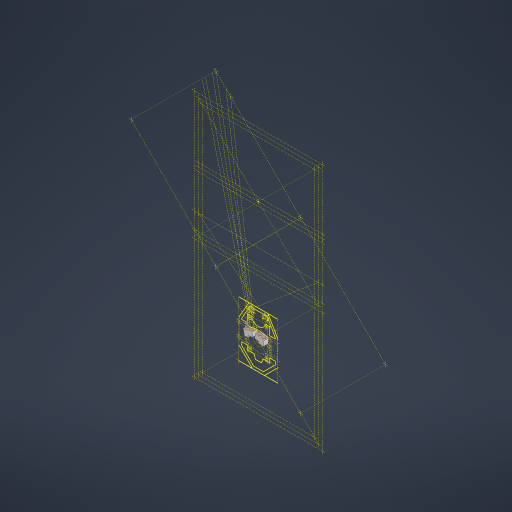
# Autodesk Inventor part: sensormount-2
Saved by Autodesk Inventor 2023.5 (Build 275446000, 446)
## iProperties
Created: 2025-01-19
Part Number: sensormount-2
Material: 一般
Document SubType Name: Modeling
Designer: IshiiLabHonda
Density: 1 g/cm^3
Appearance: 既定
Author: IshiiLabHonda
Autodesk Inventor part; units mm, degrees
(part 1 of 2)
ref_plane "YZ Plane" through (0, 0, 0) normal (1, 0, 0) x (0, 1, 0)
ref_plane "XZ Plane" through (0, 0, 0) normal (0, 1, 0) x (-1, 0, 0)
ref_plane "XY Plane" through (0, 0, 0) normal (0, 0, 1) x (1, 0, 0)
derived "chassis.ipt"
sketch "スケッチ1" plane through (0, 0, 0) normal (0, 0, 1) x (1, 0, 0)
  line L0 (-90, 90) -> (90, 90) construction
  line L1 (90, 90) -> (90, -90) construction
  line L2 (90, -90) -> (-90, -90) construction
  line L3 (-90, -90) -> (-90, 90) construction
  line L4 (-90, 90) -> (-90, 270) construction
  line L5 (-90, 270) -> (90, 270) construction
  line L6 (90, 270) -> (90, 90) construction
  line L7 (-90, 90) -> (90, -90) construction
  line L8 (90, 90) -> (-90, -90) construction
  line L9 (0, 0) -> (0, 10) construction
  line L10 (0, 0) -> (10, 0) construction
  line L11 (-90, 270) -> (90, 90) construction
  line L12 (-90, 90) -> (90, 270) construction
  line L13 (-96, 276) -> (96, 276) construction
  line L14 (96, 276) -> (96, -96) construction
  line L15 (96, -96) -> (-96, -96) construction
  line L16 (-96, -96) -> (-96, 276) construction
  line L17 (-84, 264) -> (84, 264) construction
  line L18 (84, 264) -> (84, -84) construction
  line L19 (84, -84) -> (-84, -84) construction
  line L20 (-84, -84) -> (-84, 264) construction
  line L21 (-96, 96) -> (96, 96) construction
  line L22 (-96, 84) -> (96, 84) construction
  line L23 (-63.6396, 63.6396) -> (63.6396, 190.9188) construction
  line L24 (63.6396, 190.9188) -> (190.9188, 63.6396) construction
  line L25 (190.9188, 63.6396) -> (63.6396, -63.6396) construction
  line L26 (63.6396, -63.6396) -> (-63.6396, 63.6396) construction
  line L27 (-190.9188, 190.9188) -> (-63.6396, 318.1981) construction
  line L28 (-63.6396, 318.1981) -> (63.6396, 190.9188) construction
  line L29 (-63.6396, 63.6396) -> (-190.9188, 190.9188) construction
  line L30 (-96, 120) -> (96, 120) construction
  line L31 (-96, 186) -> (96, 186) construction
  line L32 (-96, 174) -> (96, 174) construction
  line L33 (-96, 180) -> (96, 180) construction
  point P0 (-63.6396, 318.1981)
  point P1 (-90, 120)
  point P2 (90, 120)
  point P3 (0, 180)
sketch "スケッチ2" plane through (0, 0, 0) normal (0, 0, 1) x (1, 0, 0)
  line L0 (63.6396, 190.9188) -> (190.9188, 63.6396) construction
  line L1 (-63.6396, 318.1981) -> (63.6396, 190.9188) construction
  line L2 (-84, 264) -> (84, 264) construction
  line L3 (-90, 270) -> (90, 270) construction
  line L4 (90, 270) -> (90, 90) construction
  line L5 (-96, 276) -> (96, 276) construction
  line L6 (-90, 90) -> (90, 270) construction
  line L7 (-90, 270) -> (90, 90) construction
  line L8 (-63.6396, 63.6396) -> (63.6396, 190.9188) construction
  line L9 (-96, 120) -> (96, 120) construction
  line L10 (-90, 90) -> (90, 90) construction
  line L11 (-96, 96) -> (96, 96) construction
  line L12 (-96, 84) -> (96, 84) construction
  line L13 (90, -90) -> (-90, -90) construction
  line L14 (0, 0) -> (0, 10) construction
  line L15 (0, 0) -> (10, 0) construction
  line L16 (190.9188, 63.6396) -> (63.6396, -63.6396) construction
  line L17 (63.6396, -63.6396) -> (-63.6396, 63.6396) construction
  line L18 (84, -84) -> (-84, -84) construction
  line L19 (96, -96) -> (-96, -96) construction
  line L20 (-90, 90) -> (-90, 270) construction
  line L21 (-63.6396, 63.6396) -> (-190.9188, 190.9188) construction
  line L22 (-190.9188, 190.9188) -> (-63.6396, 318.1981) construction
  line L23 (96, 276) -> (96, -96) construction
  line L24 (-96, -96) -> (-96, 276) construction
  line L25 (84, 264) -> (84, -84) construction
  line L26 (-84, -84) -> (-84, 264) construction
  line L27 (90, 90) -> (90, -90) construction
  line L28 (-90, 90) -> (90, -90) construction
  line L29 (90, 90) -> (-90, -90) construction
  line L30 (-90, -90) -> (-90, 90) construction
  circle A0 centre (0, 0) radius 16 construction
  circle A1 centre (0, 0) radius 7.5 construction
  line L31 (20, 11.5) -> (28.75, 11.5) construction
  line L32 (28.75, 11.5) -> (28.75, -11.5) construction
  line L33 (28.75, -11.5) -> (20, -11.5) construction
  line L34 (20, -11.5) -> (20, 11.5) construction
  line L35 (20, 11.5) -> (18, 11.5) construction
  line L36 (18, 11.5) -> (18, -11.5) construction
  line L37 (18, -11.5) -> (20, -11.5) construction
  line L38 (18, 1.5) -> (17, 1.5) construction
  line L39 (17, -1.5) -> (18, -1.5) construction
  line L40 (-17, 26) -> (17, 26) construction
  line L41 (17, 26) -> (17, -20) construction
  line L42 (17, -20) -> (-17, -20) construction
  line L43 (-17, -20) -> (-17, 26) construction
  line L44 (-20, 11.5) -> (-18, 11.5) construction
  line L45 (-17, -1.5) -> (-18, -1.5) construction
  line L46 (-20, -11.5) -> (-20, 11.5) construction
  line L47 (-18, 11.5) -> (-18, -11.5) construction
  line L48 (-28.75, -11.5) -> (-20, -11.5) construction
  line L49 (-20, 11.5) -> (-28.75, 11.5) construction
  line L50 (-28.75, 11.5) -> (-28.75, -11.5) construction
  line L51 (-18, -11.5) -> (-20, -11.5) construction
  line L52 (-18, 1.5) -> (-17, 1.5) construction
  line L53 (-14.5, 26) -> (-14.5, -20) construction
  line L54 (14.5, 26) -> (14.5, -20) construction
  line L55 (-10.5, 26) -> (-10.5, 21) construction
  line L56 (-10.5, 21) -> (-14.5, 21) construction
  line L57 (-14.5, 26) -> (-10.5, 21) construction
  line L58 (-10.5, 26) -> (-14.5, 21) construction
  circle A2 centre (-12.5, 23.5) radius 1 construction
  line L59 (10.5, 26) -> (10.5, 21) construction
  line L60 (10.5, 21) -> (14.5, 21) construction
  line L61 (10.5, 26) -> (14.5, 21) construction
  line L62 (10.5, 21) -> (14.5, 26) construction
  circle A3 centre (12.5, 23.5) radius 1 construction
  line L63 (-14.5, -15) -> (-10.5, -15) construction
  line L64 (-10.5, -15) -> (-10.5, -20) construction
  line L65 (10.5, -20) -> (10.5, -15) construction
  line L66 (10.5, -15) -> (14.5, -15) construction
  line L67 (-14.5, -15) -> (-10.5, -20) construction
  line L68 (-10.5, -15) -> (-14.5, -20) construction
  circle A4 centre (-12.5, -17.5) radius 1 construction
  line L69 (10.5, -15) -> (14.5, -20) construction
  line L70 (14.5, -15) -> (10.5, -20) construction
  circle A5 centre (12.5, -17.5) radius 1 construction
  point P0 (90, 120)
  point P1 (-90, 120)
  point P2 (-63.6396, 318.1981)
  point P3 (-12.5, -17.5)
sketch "スケッチ3" plane through (0, 0, 0) normal (0, 0, 1) x (1, 0, 0)
  line L0 (63.6396, 190.9188) -> (190.9188, 63.6396) construction
  line L1 (-63.6396, 318.1981) -> (63.6396, 190.9188) construction
  line L2 (-84, 264) -> (84, 264) construction
  line L3 (-90, 270) -> (90, 270) construction
  line L4 (90, 270) -> (90, 90) construction
  line L5 (-96, 276) -> (96, 276) construction
  line L6 (-90, 90) -> (90, 270) construction
  line L7 (-90, 270) -> (90, 90) construction
  line L8 (-63.6396, 63.6396) -> (63.6396, 190.9188) construction
  line L9 (-96, 120) -> (96, 120) construction
  line L10 (-90, 90) -> (90, 90) construction
  line L11 (-96, 96) -> (96, 96) construction
  line L12 (-96, 84) -> (96, 84) construction
  line L13 (90, -90) -> (-90, -90) construction
  line L14 (0, 0) -> (0, 10) construction
  line L15 (0, 0) -> (10, 0) construction
  line L16 (190.9188, 63.6396) -> (63.6396, -63.6396) construction
  line L17 (63.6396, -63.6396) -> (-63.6396, 63.6396) construction
  line L18 (84, -84) -> (-84, -84) construction
  line L19 (96, -96) -> (-96, -96) construction
  line L20 (-90, 90) -> (-90, 270) construction
  line L21 (-63.6396, 63.6396) -> (-190.9188, 190.9188) construction
  line L22 (-190.9188, 190.9188) -> (-63.6396, 318.1981) construction
  line L23 (96, 276) -> (96, -96) construction
  line L24 (-96, -96) -> (-96, 276) construction
  line L25 (84, 264) -> (84, -84) construction
  line L26 (-84, -84) -> (-84, 264) construction
  line L27 (90, 90) -> (90, -90) construction
  line L28 (-90, 90) -> (90, -90) construction
  line L29 (90, 90) -> (-90, -90) construction
  line L30 (-90, -90) -> (-90, 90) construction
  line L31 (-18, 1.5) -> (-17, 1.5) construction
  line L32 (-17, -1.5) -> (-18, -1.5) construction
  line L33 (-20, 11.5) -> (-18, 11.5) construction
  line L34 (-28.75, 11.5) -> (-28.75, -11.5) construction
  line L35 (63.6396, -63.6396) -> (-63.6396, 63.6396) construction
  line L36 (84, -84) -> (-84, -84) construction
  line L37 (-90, -90) -> (-90, 90) construction
  line L38 (96, -96) -> (-96, -96) construction
  line L39 (-90, 90) -> (90, 90) construction
  line L40 (90, -90) -> (-90, -90) construction
  line L41 (90, 90) -> (-90, -90) construction
  line L42 (-90, 90) -> (90, -90) construction
  line L43 (90, 90) -> (90, -90) construction
  line L44 (-28.75, -11.5) -> (-20, -11.5) construction
  line L45 (-20, 11.5) -> (-28.75, 11.5) construction
  line L46 (-18, 11.5) -> (-18, -11.5) construction
  line L47 (-18, -11.5) -> (-20, -11.5) construction
  line L48 (0, 0) -> (0, 10) construction
  line L49 (0, 0) -> (10, 0) construction
  circle A0 centre (0, 0) radius 16 construction
  circle A1 centre (0, 0) radius 7.5 construction
  line L50 (-14.5, 26) -> (-14.5, -20) construction
  line L51 (-17, 26) -> (17, 26) construction
  line L52 (-17, -20) -> (-17, 26) construction
  line L53 (17, -20) -> (-17, -20) construction
  line L54 (-14.5, -15) -> (-10.5, -15) construction
  circle A2 centre (-12.5, -17.5) radius 1 construction
  line L55 (-10.5, -15) -> (-14.5, -20) construction
  line L56 (-14.5, -15) -> (-10.5, -20) construction
  line L57 (-63.6396, 318.1981) -> (63.6396, 190.9188) construction
  line L58 (-84, 264) -> (84, 264) construction
  line L59 (-90, 270) -> (90, 270) construction
  line L60 (90, 270) -> (90, 90) construction
  line L61 (-96, 276) -> (96, 276) construction
  line L62 (-90, 90) -> (90, 270) construction
  line L63 (-90, 270) -> (90, 90) construction
  line L64 (-63.6396, 63.6396) -> (63.6396, 190.9188) construction
  line L65 (-96, 120) -> (96, 120) construction
  line L66 (-96, 96) -> (96, 96) construction
  line L67 (-96, 84) -> (96, 84) construction
  line L68 (84, 264) -> (84, -84) construction
  line L69 (96, 276) -> (96, -96) construction
  line L70 (-96, -96) -> (-96, 276) construction
  line L71 (-84, -84) -> (-84, 264) construction
  line L72 (-63.6396, 63.6396) -> (-190.9188, 190.9188) construction
  line L73 (-90, 90) -> (-90, 270) construction
  line L74 (-190.9188, 190.9188) -> (-63.6396, 318.1981) construction
  line L75 (-20, -11.5) -> (-20, 11.5) construction
  line L76 (10.5, -15) -> (14.5, -15) construction
  line L77 (10.5, -20) -> (10.5, -15) construction
  circle A3 centre (12.5, -17.5) radius 1 construction
  line L78 (10.5, -15) -> (14.5, -20) construction
  line L79 (14.5, -15) -> (10.5, -20) construction
  line L80 (-10.5, -15) -> (-10.5, -20) construction
  line L81 (63.6396, 190.9188) -> (190.9188, 63.6396) construction
  line L82 (190.9188, 63.6396) -> (63.6396, -63.6396) construction
  line L83 (20, 11.5) -> (28.75, 11.5) construction
  line L84 (28.75, 11.5) -> (28.75, -11.5) construction
  line L85 (17, -1.5) -> (18, -1.5) construction
  line L86 (18, -11.5) -> (20, -11.5) construction
  line L87 (28.75, -11.5) -> (20, -11.5) construction
  line L88 (14.5, 26) -> (14.5, -20) construction
  line L89 (17, 26) -> (17, -20) construction
  line L90 (18, 11.5) -> (18, -11.5) construction
  line L91 (20, -11.5) -> (20, 11.5) construction
  line L92 (20, 11.5) -> (18, 11.5) construction
  line L93 (18, 1.5) -> (17, 1.5) construction
  line L94 (-10.5, 26) -> (-10.5, 21) construction
  line L95 (10.5, 21) -> (14.5, 21) construction
  circle A4 centre (12.5, 23.5) radius 1 construction
  line L96 (10.5, 26) -> (14.5, 21) construction
  line L97 (10.5, 21) -> (14.5, 26) construction
  line L98 (10.5, 26) -> (10.5, 21) construction
  line L99 (-10.5, 21) -> (-14.5, 21) construction
  circle A5 centre (-12.5, 23.5) radius 1 construction
  line L100 (-14.5, 26) -> (-10.5, 21) construction
  line L101 (-10.5, 26) -> (-14.5, 21) construction
  line L102 (29.25, 41.8164) -> (29.25, -41.1836) construction
  line L103 (29.25, -41.1836) -> (-29.25, -41.1836) construction
  line L104 (-29.25, -41.1836) -> (-29.25, 41.8164) construction
  line L105 (-29.25, 8.5) -> (-17, 8.5) construction
  line L106 (-17, 8.5) -> (-17, -8.5) construction
  line L107 (-17, -8.5) -> (-29.25, -8.5) construction
  line L108 (29.25, 8.5) -> (17, 8.5) construction
  line L109 (17, 8.5) -> (17, -8.5) construction
  line L110 (17, -8.5) -> (29.25, -8.5) construction
  line L111 (-2.6232, 12.9386) -> (-1.1431, 4.3146) construction
  line L112 (6.5255, 35.7419) -> (9.7395, 39.5722) construction
  line L113 (5.3082, 35.458) -> (9.8077, 40.8203) construction
  line L114 (10.2875, 31.2799) -> (5.3082, 35.458) construction
  line L115 (9.8077, 40.8203) -> (10.2875, 31.2799) construction
  line L116 (10.3558, 32.528) -> (9.7395, 39.5722) construction
  line L117 (10.3558, 32.528) -> (6.5255, 35.7419) construction
  line L118 (10.2875, 31.2799) -> (12.5856, 29.3515) construction
  line L119 (9.7395, 39.5722) -> (13.5697, 36.3582) construction
  line L120 (6.5255, 35.7419) -> (13.5697, 36.3582) construction
  line L121 (13.5697, 36.3582) -> (10.3558, 32.528) construction
  line L122 (5.3082, 35.458) -> (14.787, 36.6422) construction
  line L123 (9.8077, 40.8203) -> (14.787, 36.6422) construction
  line L124 (14.787, 36.6422) -> (10.2875, 31.2799) construction
  line L125 (12.5856, 29.3515) -> (17.0851, 34.7138) construction
  line L126 (17.0851, 34.7138) -> (14.787, 36.6422) construction
  line L127 (-3.4819, 12.0302) -> (-2.6362, 7.1023) construction
  line L128 (-8.4099, 11.1845) -> (-2.6362, 7.1023) construction
  line L129 (-7.5641, 6.2565) -> (-3.4819, 12.0302) construction
  line L130 (-9.0295, 11.8391) -> (-2.6232, 12.9386) construction
  line L131 (-7.5641, 6.2565) -> (-8.4099, 11.1845) construction
  line L132 (-1.1431, 4.3146) -> (-7.5495, 3.2152) construction
  line L133 (-7.5495, 3.2152) -> (-9.0295, 11.8391) construction
  line L134 (-63.6396, 318.1981) -> (-5.523, 9.1434) construction
  line L135 (10.0476, 36.0501) -> (-90, 120) construction
  line L136 (-5.523, 9.1434) -> (-79.4519, 302.3857) construction
  line L137 (-5.523, 9.1434) -> (-41.5159, 296.0744) construction
  line L138 (-10.0476, 36.0501) -> (90, 120) construction
  line L139 (-9.7395, 39.5722) -> (-6.5255, 35.7419) construction
  line L140 (-9.8077, 40.8203) -> (-5.3082, 35.458) construction
  line L141 (-14.787, 36.6422) -> (-9.8077, 40.8203) construction
  line L142 (-5.3082, 35.458) -> (-14.787, 36.6422) construction
  line L143 (-13.5697, 36.3582) -> (-6.5255, 35.7419) construction
  line L144 (-13.5697, 36.3582) -> (-9.7395, 39.5722) construction
  line L145 (-14.787, 36.6422) -> (-17.0851, 34.7138) construction
  line L146 (-6.5255, 35.7419) -> (-10.3558, 32.528) construction
  line L147 (-9.7395, 39.5722) -> (-10.3558, 32.528) construction
  line L148 (-9.8077, 40.8203) -> (-10.2875, 31.2799) construction
  line L149 (-5.3082, 35.458) -> (-10.2875, 31.2799) construction
  line L150 (-10.2875, 31.2799) -> (-14.787, 36.6422) construction
  line L151 (-17.0851, 34.7138) -> (-12.5856, 29.3515) construction
  line L152 (-12.5856, 29.3515) -> (-10.2875, 31.2799) construction
  line L153 (-10.3558, 32.528) -> (-13.5697, 36.3582) construction
  circle A6 centre (-6.8337, 32.2199) radius 0.625 construction
  circle A7 centre (-6.8337, 32.2199) radius 0.8 construction
  circle A8 centre (-6.8337, 32.2199) radius 1.5 construction
  circle A9 centre (-13.6863, 32.9968) radius 1.5 construction
  circle A10 centre (-13.6863, 32.9968) radius 0.8 construction
  circle A11 centre (-13.6863, 32.9968) radius 0.625 construction
  line L154 (-2.6362, 7.1023) -> (-7.5641, 6.2565) construction
  line L155 (-7.9301, 5.4327) -> (-1.5237, 6.5322) construction
  line L156 (-7.987, 8.7205) -> (-3.059, 9.5662) construction
  line L157 (-4.5927, 3.7226) -> (-5.1001, 6.6794) construction
  line L158 (-8.4099, 11.1845) -> (-3.4819, 12.0302) construction
  circle A12 centre (13.6863, 32.9968) radius 1.5 construction
  circle A13 centre (13.6863, 32.9968) radius 0.625 construction
  circle A14 centre (13.6863, 32.9968) radius 0.8
  circle A15 centre (6.8337, 32.2199) radius 1.5 construction
  circle A16 centre (6.8337, 32.2199) radius 0.8
  circle A17 centre (6.8337, 32.2199) radius 0.625 construction
  line L159 (-29.25, -41.1836) -> (29.25, -41.1836)
  line L160 (-29.25, 41.8164) -> (29.25, 41.8164)
  line L161 (-10.0476, 36.0501) -> (-6.8337, 32.2199) construction
  line L162 (-29.25, 15.7886) -> (-14.2228, 41.8164)
  line L163 (-29.25, -20.8975) -> (-8.9639, -41.1836)
  line L164 (29.25, 15.7886) -> (14.2228, 41.8164)
  line L165 (29.25, -20.8975) -> (8.9639, -41.1836)
  line L166 (25.25, 15.774) -> (25.25, 14.5)
  line L167 (25.25, 14.5) -> (17, 14.5)
  line L168 (3.695, 18.0905) -> (-3.695, 18.0905)
  line L169 (-17, 14.5) -> (-25.25, 14.5)
  line L170 (-25.25, 14.5) -> (-25.25, 15.774)
  line L171 (1.1431, 4.3146) -> (7.5495, 3.2152) construction
  line L172 (7.5495, 3.2152) -> (9.0295, 11.8391) construction
  line L173 (2.6232, 12.9386) -> (1.1431, 4.3146) construction
  line L174 (2.6362, 7.1023) -> (7.5641, 6.2565) construction
  line L175 (7.9301, 5.4327) -> (1.5237, 6.5322) construction
  line L176 (8.4099, 11.1845) -> (2.6362, 7.1023) construction
  line L177 (7.5641, 6.2565) -> (3.4819, 12.0302) construction
  line L178 (3.4819, 12.0302) -> (2.6362, 7.1023) construction
  line L179 (8.4099, 11.1845) -> (3.4819, 12.0302) construction
  line L180 (7.5641, 6.2565) -> (8.4099, 11.1845) construction
  line L181 (9.0295, 11.8391) -> (2.6232, 12.9386) construction
  line L182 (-9.7365, 22.9366) -> (-9.7365, 26)
  line L183 (9.7365, 22.9366) -> (9.7365, 26)
  line L184 (9.7365, 26) -> (17, 26)
  line L185 (17, 26) -> (17, 14.5)
  line L186 (-9.7365, 26) -> (-17, 26)
  line L187 (-17, 26) -> (-17, 14.5)
  line L188 (-9.7365, 22.9366) -> (-3.695, 18.0905)
  line L189 (9.7365, 22.9366) -> (3.695, 18.0905)
  line L190 (-17, -14.5) -> (-25.25, -14.5)
  line L191 (-25.25, -14.5) -> (-25.25, -19.2406)
  line L192 (-25.25, -19.2406) -> (-7.307, -37.1836)
  line L193 (-7.307, -37.1836) -> (7.307, -37.1836)
  line L194 (7.307, -37.1836) -> (25.25, -19.2406)
  line L195 (25.25, -19.2406) -> (25.25, -14.5)
  line L196 (25.25, -14.5) -> (17, -14.5)
  line L197 (17, -14.5) -> (17, -20.8804)
  line L198 (17, -20.8804) -> (6.6466, -20.8804)
  line L199 (6.6466, -20.8804) -> (4.5158, -27.0126)
  line L200 (4.5158, -27.0126) -> (-4.5158, -27.0126)
  line L201 (-4.5158, -27.0126) -> (-6.6466, -20.8804)
  line L202 (-6.6466, -20.8804) -> (-17, -20.8804)
  line L203 (-17, -20.8804) -> (-17, -14.5)
  line L204 (-9.0295, 11.8391) -> (-7.5495, 3.2152) construction
  line L205 (-9.3955, 11.0153) -> (-8.5497, 6.0874) construction
  line L206 (-14.3234, 10.1696) -> (-8.5497, 6.0874) construction
  line L207 (-13.4777, 5.2416) -> (-9.3955, 11.0153) construction
  line L208 (-13.4777, 5.2416) -> (-14.3234, 10.1696) construction
  line L209 (-7.5495, 3.2152) -> (-13.9558, 2.1157) construction
  line L210 (-13.9558, 2.1157) -> (-15.4359, 10.7396) construction
  line L211 (-14.3234, 10.1696) -> (-9.3955, 11.0153) construction
  line L212 (-13.9005, 7.7056) -> (-8.9726, 8.5513) construction
  line L213 (-8.5497, 6.0874) -> (-13.4777, 5.2416) construction
  line L214 (-10.5062, 2.7077) -> (-11.0137, 5.6645) construction
  line L215 (-15.4359, 10.7396) -> (-9.0295, 11.8391) construction
  line L216 (9.3955, 11.0153) -> (8.5497, 6.0874) construction
  line L217 (9.0295, 11.8391) -> (7.5495, 3.2152) construction
  line L218 (14.3234, 10.1696) -> (9.3955, 11.0153) construction
  line L219 (13.9005, 7.7056) -> (8.9726, 8.5513) construction
  line L220 (10.5062, 2.7077) -> (11.0137, 5.6645) construction
  line L221 (15.4359, 10.7396) -> (9.0295, 11.8391) construction
  line L222 (13.4777, 5.2416) -> (9.3955, 11.0153) construction
  line L223 (8.5497, 6.0874) -> (13.4777, 5.2416) construction
  line L224 (14.3234, 10.1696) -> (8.5497, 6.0874) construction
  line L225 (13.4777, 5.2416) -> (14.3234, 10.1696) construction
  line L226 (13.9558, 2.1157) -> (15.4359, 10.7396) construction
  line L227 (7.5495, 3.2152) -> (13.9558, 2.1157) construction
  line L228 (14.1851, 3.4517) -> (7.8081, 4.722) construction
  line L229 (-25.25, 15.774) -> (-13.111, 37.7059)
  line L230 (-13.111, 37.7059) -> (13.111, 37.7059)
  line L231 (13.111, 37.7059) -> (25.25, 15.774)
  circle A18 centre (0, 0) radius 4.25 construction
  line L232 (-11.4366, 8.1285) -> (-68.7778, 313.0599) construction
  line L233 (-11.4366, 8.1285) -> (-84.3791, 297.4585) construction
  line L234 (-11.4366, 8.1285) -> (-48.4232, 302.9817) construction
  line L235 (-15.4359, 10.7396) -> (-13.9558, 2.1157) construction
  line L236 (-14.3364, 4.3333) -> (-7.9301, 5.4327) construction
  point P0 (-7.5593, 4.6422)
  point P1 (25.25, 25.1515)
  point P2 (11.4366, 8.1285)
  point P3 (11.4366, 8.1285)
  point P4 (-5.523, 9.1434)
  point P5 (-5.523, 9.1434)
sketch "スケッチ4" plane through (0, 0, 0) normal (0, 0, 1) x (1, 0, 0)
  line L0 (-90, 90) -> (90, 90) construction
  line L1 (90, 90) -> (90, -90) construction
  line L2 (90, -90) -> (-90, -90) construction
  line L3 (-90, -90) -> (-90, 90) construction
  line L4 (0, 0) -> (0, 10) construction
  line L5 (0, 0) -> (10, 0) construction
  line L6 (63.6396, -63.6396) -> (-63.6396, 63.6396) construction
  line L7 (-90, 90) -> (90, -90) construction
  line L8 (90, 90) -> (-90, -90) construction
  line L9 (84, -84) -> (-84, -84) construction
  line L10 (96, -96) -> (-96, -96) construction
  line L11 (-90, 270) -> (90, 270) construction
  line L12 (-84, 264) -> (84, 264) construction
  line L13 (-63.6396, 318.1981) -> (63.6396, 190.9188) construction
  line L14 (-96, 276) -> (96, 276) construction
  line L15 (-90, 90) -> (-90, 270) construction
  line L16 (-96, 84) -> (96, 84) construction
  line L17 (-96, 96) -> (96, 96) construction
  line L18 (-96, 120) -> (96, 120) construction
  line L19 (96, 276) -> (96, -96) construction
  line L20 (-96, -96) -> (-96, 276) construction
  line L21 (-84, -84) -> (-84, 264) construction
  line L22 (84, 264) -> (84, -84) construction
  line L23 (-63.6396, 63.6396) -> (63.6396, 190.9188) construction
  line L24 (-96, 180) -> (96, 180) construction
  line L25 (-96, 186) -> (96, 186) construction
  line L26 (-90, 270) -> (90, 90) construction
  line L27 (90, 270) -> (90, 90) construction
  line L28 (-90, 90) -> (90, 270) construction
  line L29 (-96, 174) -> (96, 174) construction
  line L30 (-190.9188, 190.9188) -> (-63.6396, 318.1981) construction
  line L31 (-63.6396, 63.6396) -> (-190.9188, 190.9188) construction
  line L32 (63.6396, 190.9188) -> (190.9188, 63.6396) construction
  line L33 (190.9188, 63.6396) -> (63.6396, -63.6396) construction
  line L34 (-63.6396, 63.6396) -> (-190.9188, 190.9188) construction
  line L35 (-90, 90) -> (-90, 270) construction
  line L36 (-190.9188, 190.9188) -> (-63.6396, 318.1981) construction
  line L37 (0, 0) -> (0, 10) construction
  line L38 (-10.5, 21) -> (-14.5, 21) construction
  circle A0 centre (0, 0) radius 7.5 construction
  line L39 (-10.5, 26) -> (-14.5, 21) construction
  line L40 (-14.5, 26) -> (-10.5, 21) construction
  line L41 (0, 0) -> (10, 0) construction
  line L42 (-17, -20) -> (-17, 26) construction
  circle A1 centre (0, 0) radius 16 construction
  line L43 (-14.5, 26) -> (-14.5, -20) construction
  line L44 (17, -20) -> (-17, -20) construction
  line L45 (14.5, 26) -> (14.5, -20) construction
  line L46 (17, 26) -> (17, -20) construction
  line L47 (18, 11.5) -> (18, -11.5) construction
  line L48 (20, -11.5) -> (20, 11.5) construction
  line L49 (-18, 11.5) -> (-18, -11.5) construction
  line L50 (-20, -11.5) -> (-20, 11.5) construction
  line L51 (-17, -1.5) -> (-18, -1.5) construction
  line L52 (-20, 11.5) -> (-18, 11.5) construction
  line L53 (-18, 1.5) -> (-17, 1.5) construction
  line L54 (190.9188, 63.6396) -> (63.6396, -63.6396) construction
  line L55 (20, 11.5) -> (28.75, 11.5) construction
  line L56 (28.75, 11.5) -> (28.75, -11.5) construction
  line L57 (17, -1.5) -> (18, -1.5) construction
  line L58 (18, 1.5) -> (17, 1.5) construction
  line L59 (20, 11.5) -> (18, 11.5) construction
  circle A2 centre (-12.5, 23.5) radius 1 construction
  line L60 (-18, -11.5) -> (-20, -11.5) construction
  line L61 (63.6396, 190.9188) -> (190.9188, 63.6396) construction
  line L62 (-63.6396, 318.1981) -> (63.6396, 190.9188) construction
  line L63 (-84, 264) -> (84, 264) construction
  line L64 (-90, 270) -> (90, 270) construction
  line L65 (90, 270) -> (90, 90) construction
  line L66 (-96, 276) -> (96, 276) construction
  line L67 (-20, 11.5) -> (-28.75, 11.5) construction
  line L68 (-63.6396, 63.6396) -> (63.6396, 190.9188) construction
  line L69 (-28.75, 11.5) -> (-28.75, -11.5) construction
  line L70 (-28.75, -11.5) -> (-20, -11.5) construction
  line L71 (-90, 90) -> (90, 270) construction
  line L72 (-90, 270) -> (90, 90) construction
  line L73 (-90, 90) -> (90, 90) construction
  line L74 (-96, 120) -> (96, 120) construction
  line L75 (-96, 96) -> (96, 96) construction
  line L76 (-96, 84) -> (96, 84) construction
  line L77 (-84, -84) -> (-84, 264) construction
  line L78 (-96, -96) -> (-96, 276) construction
  line L79 (84, 264) -> (84, -84) construction
  line L80 (96, 276) -> (96, -96) construction
  line L81 (-90, -90) -> (-90, 90) construction
  line L82 (63.6396, -63.6396) -> (-63.6396, 63.6396) construction
  line L83 (84, -84) -> (-84, -84) construction
  line L84 (90, -90) -> (-90, -90) construction
  line L85 (90, 90) -> (90, -90) construction
  line L86 (-90, 90) -> (90, -90) construction
  line L87 (96, -96) -> (-96, -96) construction
  line L88 (90, 90) -> (-90, -90) construction
  line L89 (10.5, 26) -> (10.5, 21) construction
  line L90 (10.5, 21) -> (14.5, 21) construction
  circle A3 centre (12.5, 23.5) radius 1 construction
  line L91 (10.5, 21) -> (14.5, 26) construction
  line L92 (10.5, 26) -> (14.5, 21) construction
  line L93 (-10.5, 26) -> (-10.5, 21) construction
  line L94 (28.75, -11.5) -> (20, -11.5) construction
  line L95 (18, -11.5) -> (20, -11.5) construction
  circle A4 centre (12.5, -17.5) radius 1 construction
  line L96 (-14.5, -15) -> (-10.5, -15) construction
  circle A5 centre (-12.5, -17.5) radius 1 construction
  line L97 (-14.5, -15) -> (-10.5, -20) construction
  line L98 (-10.5, -15) -> (-14.5, -20) construction
  line L99 (-10.5, -15) -> (-10.5, -20) construction
  line L100 (10.5, -15) -> (14.5, -15) construction
  line L101 (10.5, -20) -> (10.5, -15) construction
  line L102 (10.5, -15) -> (14.5, -20) construction
  line L103 (14.5, -15) -> (10.5, -20) construction
  line L104 (-96, 96) -> (96, 96) construction
  line L105 (-96, 84) -> (96, 84) construction
  line L106 (-96, 84) -> (96, 84) construction
  line L107 (96, -96) -> (-96, -96) construction
  line L108 (96, -96) -> (-96, -96) construction
  line L109 (-96, 96) -> (96, 96) construction
  circle A6 centre (-6.8337, 32.2199) radius 1.5 construction
  line L110 (-20, 11.5) -> (-28.75, 11.5) construction
  line L111 (-20, 11.5) -> (-18, 11.5) construction
  line L112 (-18, 1.5) -> (-17, 1.5) construction
  line L113 (-28.75, 11.5) -> (-28.75, -11.5) construction
  line L114 (-28.75, -11.5) -> (-20, -11.5) construction
  line L115 (63.6396, -63.6396) -> (-63.6396, 63.6396) construction
  line L116 (63.6396, -63.6396) -> (-63.6396, 63.6396) construction
  line L117 (-90, 90) -> (90, 90) construction
  line L118 (-90, 90) -> (90, 90) construction
  line L119 (-90, -90) -> (-90, 90) construction
  line L120 (-90, -90) -> (-90, 90) construction
  line L121 (90, 90) -> (90, -90) construction
  line L122 (90, 90) -> (90, -90) construction
  line L123 (90, 90) -> (-90, -90) construction
  line L124 (90, 90) -> (-90, -90) construction
  line L125 (-90, 90) -> (90, -90) construction
  line L126 (-90, 90) -> (90, -90) construction
  line L127 (84, -84) -> (-84, -84) construction
  line L128 (90, -90) -> (-90, -90) construction
  line L129 (90, -90) -> (-90, -90) construction
  line L130 (84, -84) -> (-84, -84) construction
  line L131 (-84, 264) -> (84, 264) construction
  line L132 (-90, 90) -> (90, 270) construction
  line L133 (-90, 90) -> (90, 270) construction
  line L134 (-84, 264) -> (84, 264) construction
  line L135 (-13.5697, 36.3582) -> (-6.5255, 35.7419) construction
  line L136 (-17, -1.5) -> (-18, -1.5) construction
  circle A7 centre (-6.8337, 32.2199) radius 0.8 construction
  line L137 (-13.5697, 36.3582) -> (-9.7395, 39.5722) construction
  circle A8 centre (-13.6863, 32.9968) radius 0.625 construction
  line L138 (-17, -20) -> (-17, 26) construction
  circle A9 centre (-13.6863, 32.9968) radius 0.8 construction
  circle A10 centre (-13.6863, 32.9968) radius 1.5 construction
  line L139 (-17.0851, 34.7138) -> (-12.5856, 29.3515) construction
  line L140 (-14.787, 36.6422) -> (-17.0851, 34.7138) construction
  line L141 (-10.2875, 31.2799) -> (-14.787, 36.6422) construction
  line L142 (-10.3558, 32.528) -> (-13.5697, 36.3582) construction
  line L143 (-8.4099, 11.1845) -> (-3.4819, 12.0302) construction
  line L144 (-3.4819, 12.0302) -> (-2.6362, 7.1023) construction
  line L145 (-4.5927, 3.7226) -> (-5.1001, 6.6794) construction
  line L146 (-7.5641, 6.2565) -> (-3.4819, 12.0302) construction
  line L147 (-8.4099, 11.1845) -> (-2.6362, 7.1023) construction
  line L148 (-2.6362, 7.1023) -> (-7.5641, 6.2565) construction
  line L149 (-7.5641, 6.2565) -> (-8.4099, 11.1845) construction
  line L150 (-7.987, 8.7205) -> (-3.059, 9.5662) construction
  line L151 (0, 0) -> (0, 10) construction
  line L152 (0, 0) -> (10, 0) construction
  line L153 (-18, 11.5) -> (-18, -11.5) construction
  line L154 (-18, -11.5) -> (-20, -11.5) construction
  line L155 (0, 0) -> (0, 10) construction
  line L156 (0, 0) -> (10, 0) construction
  circle A11 centre (0, 0) radius 16 construction
  circle A12 centre (0, 0) radius 7.5 construction
  line L157 (17, -20) -> (-17, -20) construction
  line L158 (-14.5, 26) -> (-14.5, -20) construction
  line L159 (-9.0295, 11.8391) -> (-2.6232, 12.9386) projected
  line L160 (-10.5, 21) -> (-14.5, 21) construction
  line L161 (-10.5, 26) -> (-10.5, 21) construction
  circle A13 centre (-12.5, 23.5) radius 1 construction
  line L162 (-14.5, 26) -> (-10.5, 21) construction
  line L163 (-29.25, 8.5) -> (-17, 8.5) construction
  line L164 (-10.5, 26) -> (-14.5, 21) construction
  line L165 (12.5856, 29.3515) -> (17.0851, 34.7138) construction
  line L166 (-2.6232, 12.9386) -> (-1.1431, 4.3146) projected
  line L167 (-1.1431, 4.3146) -> (-7.5495, 3.2152) projected
  line L168 (-7.9301, 5.4327) -> (-1.5237, 6.5322) projected
  line L169 (-7.5495, 3.2152) -> (-9.0295, 11.8391) projected
  line L170 (-5.3082, 35.458) -> (-14.787, 36.6422) construction
  line L171 (-14.787, 36.6422) -> (-9.8077, 40.8203) construction
  line L172 (-20, -11.5) -> (-20, 11.5) construction
  line L173 (10.5, -15) -> (14.5, -15) construction
  line L174 (-17, 8.5) -> (-17, -8.5) construction
  line L175 (-17, -8.5) -> (-29.25, -8.5) construction
  line L176 (-10.5, -15) -> (-10.5, -20) construction
  line L177 (20, 11.5) -> (18, 11.5) construction
  line L178 (18, 1.5) -> (17, 1.5) construction
  line L179 (17, -1.5) -> (18, -1.5) construction
  line L180 (18, 11.5) -> (18, -11.5) construction
  line L181 (18, -11.5) -> (20, -11.5) construction
  line L182 (10.5, -20) -> (10.5, -15) construction
  circle A14 centre (12.5, -17.5) radius 1 construction
  line L183 (10.5, -15) -> (14.5, -20) construction
  line L184 (14.5, -15) -> (10.5, -20) construction
  line L185 (-29.25, -41.1836) -> (-29.25, 41.8164) construction
  line L186 (29.25, -41.1836) -> (-29.25, -41.1836) construction
  line L187 (14.5, 26) -> (14.5, -20) construction
  line L188 (17, 26) -> (17, -20) construction
  line L189 (28.75, 11.5) -> (28.75, -11.5) construction
  line L190 (28.75, -11.5) -> (20, -11.5) construction
  line L191 (17, 8.5) -> (17, -8.5) construction
  line L192 (-63.6396, 63.6396) -> (63.6396, 190.9188) construction
  line L193 (-63.6396, 63.6396) -> (63.6396, 190.9188) construction
  line L194 (-63.6396, 318.1981) -> (63.6396, 190.9188) construction
  line L195 (-90, 270) -> (90, 270) construction
  line L196 (90, 270) -> (90, 90) construction
  line L197 (-96, 120) -> (96, 120) construction
  line L198 (-96, 120) -> (96, 120) construction
  line L199 (10.0476, 36.0501) -> (-90, 120) construction
  line L200 (-96, -96) -> (-96, 276) construction
  line L201 (-96, -96) -> (-96, 276) construction
  line L202 (96, 276) -> (96, -96) construction
  line L203 (96, 276) -> (96, -96) construction
  line L204 (-84, -84) -> (-84, 264) construction
  line L205 (-84, -84) -> (-84, 264) construction
  line L206 (84, 264) -> (84, -84) construction
  line L207 (84, 264) -> (84, -84) construction
  line L208 (-90, 90) -> (-90, 270) construction
  line L209 (-90, 90) -> (-90, 270) construction
  line L210 (-90, 270) -> (90, 90) construction
  line L211 (-90, 270) -> (90, 90) construction
  line L212 (90, 270) -> (90, 90) construction
  line L213 (-5.523, 9.1434) -> (-41.5159, 296.0744) construction
  line L214 (-5.523, 9.1434) -> (-79.4519, 302.3857) construction
  line L215 (-63.6396, 318.1981) -> (-5.523, 9.1434) construction
  line L216 (-90, 270) -> (90, 270) construction
  line L217 (-96, 276) -> (96, 276) construction
  line L218 (-96, 276) -> (96, 276) construction
  line L219 (-63.6396, 318.1981) -> (63.6396, 190.9188) construction
  line L220 (-63.6396, 63.6396) -> (-190.9188, 190.9188) construction
  line L221 (-63.6396, 63.6396) -> (-190.9188, 190.9188) construction
  line L222 (-190.9188, 190.9188) -> (-63.6396, 318.1981) construction
  line L223 (-190.9188, 190.9188) -> (-63.6396, 318.1981) construction
  line L224 (-14.5, -15) -> (-10.5, -15) construction
  circle A15 centre (-12.5, -17.5) radius 1 construction
  line L225 (-14.5, -15) -> (-10.5, -20) construction
  line L226 (-10.5, -15) -> (-14.5, -20) construction
  line L227 (9.7395, 39.5722) -> (13.5697, 36.3582) construction
  line L228 (6.5255, 35.7419) -> (13.5697, 36.3582) construction
  line L229 (-9.7395, 39.5722) -> (-6.5255, 35.7419) construction
  line L230 (5.3082, 35.458) -> (14.787, 36.6422) construction
  line L231 (-9.8077, 40.8203) -> (-5.3082, 35.458) construction
  line L232 (17.0851, 34.7138) -> (14.787, 36.6422) construction
  line L233 (10.3558, 32.528) -> (9.7395, 39.5722) construction
  line L234 (10.3558, 32.528) -> (6.5255, 35.7419) construction
  line L235 (13.5697, 36.3582) -> (10.3558, 32.528) construction
  line L236 (14.787, 36.6422) -> (10.2875, 31.2799) construction
  line L237 (9.8077, 40.8203) -> (10.2875, 31.2799) construction
  line L238 (10.2875, 31.2799) -> (5.3082, 35.458) construction
  circle A16 centre (-6.8337, 32.2199) radius 0.625 construction
  line L239 (-6.5255, 35.7419) -> (-10.3558, 32.528) construction
  line L240 (-9.7395, 39.5722) -> (-10.3558, 32.528) construction
  line L241 (-9.8077, 40.8203) -> (-10.2875, 31.2799) construction
  line L242 (-5.3082, 35.458) -> (-10.2875, 31.2799) construction
  line L243 (6.5255, 35.7419) -> (9.7395, 39.5722) construction
  line L244 (5.3082, 35.458) -> (9.8077, 40.8203) construction
  line L245 (20, -11.5) -> (20, 11.5) construction
  line L246 (20, 11.5) -> (28.75, 11.5) construction
  line L247 (10.5, 21) -> (14.5, 21) construction
  line L248 (10.5, 26) -> (14.5, 21) construction
  line L249 (10.5, 21) -> (14.5, 26) construction
  line L250 (10.5, 26) -> (10.5, 21) construction
  line L251 (17, -8.5) -> (29.25, -8.5) construction
  circle A17 centre (12.5, 23.5) radius 1 construction
  line L252 (-10.0476, 36.0501) -> (90, 120) construction
  line L253 (63.6396, 190.9188) -> (190.9188, 63.6396) construction
  line L254 (63.6396, 190.9188) -> (190.9188, 63.6396) construction
  line L255 (9.8077, 40.8203) -> (14.787, 36.6422) construction
  line L256 (190.9188, 63.6396) -> (63.6396, -63.6396) construction
  line L257 (190.9188, 63.6396) -> (63.6396, -63.6396) construction
  line L258 (29.25, 8.5) -> (17, 8.5) construction
  circle A18 centre (6.8337, 32.2199) radius 0.625 construction
  circle A19 centre (6.8337, 32.2199) radius 0.8 projected
  circle A20 centre (13.6863, 32.9968) radius 0.625 construction
  circle A21 centre (13.6863, 32.9968) radius 0.8 projected
  circle A22 centre (13.6863, 32.9968) radius 1.5 construction
  line L259 (-15.4359, 10.7396) -> (-9.0295, 11.8391) projected
  line L260 (-13.9558, 2.1157) -> (-15.4359, 10.7396) projected
  line L261 (-7.5495, 3.2152) -> (-13.9558, 2.1157) projected
  line L262 (-14.3364, 4.3333) -> (-7.9301, 5.4327) projected
  point P0 (0, 180)
  point P1 (-12.5, -17.5)
  point P2 (-7.5593, 4.6422)
  point P3 (-1.5237, 6.5322)
  constraints: 68 other
extrude "押し出し7" add sketch "スケッチ4" along normal blind 7 contours L159 L166 L168 L169 | L169 L262 L260 L259 | L168 L166 L167 L169 | L169 L261 L260 L262
ref_plane "作業平面3" through (-15.4359, 10.7396, 7) normal (-0.1691495, 0.9855904, 0) x (0.9855904, 0.1691495, 0)
sketch "スケッチ6" plane through (-15.4359, 10.7396, 7) normal (-0.1691495, 0.9855904, 0) x (0.9855904, 0.1691495, 0)
  line L0 (13, 7) -> (0, 7) projected
  line L1 (0, 7) -> (0, 0) projected
  line L2 (13, 0) -> (0, 0) projected
  line L3 (13, 7) -> (13, 0) projected
  line L4 (7, 0) -> (7, 7) construction
  line L5 (6, 0) -> (6, 7) construction
  line L6 (12, 0) -> (12, 7) construction
  line L7 (1, 0) -> (1, 7) construction
  line L8 (13, 0) -> (0, 0) projected
  line L9 (13, 7) -> (0, 7) projected
  line L10 (13, 6) -> (0, 6) construction
  line L11 (13, 1) -> (0, 1) construction
  line L12 (0, 7) -> (0, 0) projected
  line L13 (12, 1) -> (7, 6) construction
  line L14 (12, 6) -> (7, 1) construction
  line L15 (6, 1) -> (1, 6) construction
  line L16 (6, 6) -> (1, 1) construction
  circle A0 centre (9.5, 3.5) radius 2.5
  circle A1 centre (3.5, 3.5) radius 2.5
  point P0 (13.3968, 7)
  dimension "d22" = 1
  dimension "d23" = 5
  dimension "d24" = 1
  dimension "d25" = 5
  dimension "d26" = 1
  dimension "d27" = 1
  dimension "d28" = 5
  dimension "d29" = 5
  constraints: 28 point on line, 20 end point, 6 parallel, 2 centre point, 2 midpoint, 1 perpendicular
  measures "d22" distance between parallel lines of L3 L6
  measures "d23" distance between parallel lines of L6 L4
  measures "d24" distance between parallel lines of L4 L5
  measures "d25" distance between parallel lines of L5 L7
  measures "d26" distance between parallel lines of L0 L10
  measures "d27" distance between parallel lines of L2 L11
  measures "d28" diameter of A0
  measures "d29" diameter of A1
extrude "押し出し8" cut sketch "スケッチ6" against normal blind 10 contours A0 | A1
mirror "ミラー2" about plane through (0, 0, 0) normal (1, 0, 0) of "押し出し8", "押し出し7"